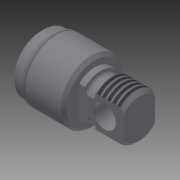
# Autodesk Inventor part: D-15705rear_head
Saved by Autodesk Inventor 2014 (Build 180170000, 170)
## iProperties
Created: 2014-01-19
Part Number: D-15705rear_head
Material: Steel
Catalog Web Link: www.cadenas.de
Description: Rear Head Cyl-Original Line Cyl
Vendor: BIMBA
Document SubType Name: Standard Catalog Part
Designer: Michael
Manufacturer: BIMBA
Density: 7.85 g/cm^3
Appearance: Steel
Mass: 19.7637 g
Surface Area: 18.1502 cm^2
Volume: 2.51767 cm^3
Category: PARTsolutions
Company: BIMBA
PSOL_IDENT_0: {$CADENAS_DATA\23d-libs\bimba\bimba\bimba_imperial\bimba_full_line\original_line_cylinders\three_pos
PSOL_IDENT_1: ition_cylinders\rear_head_cyl.prj},185 {VTYP=3D},{NB=D-15705rear_head},{LINA=D-15705rear_head},{NN=R
PSOL_IDENT_2: ear Head Cyl},{DATE=20.08.2011 07:16:50},{GEOMDATE=02.08.2011 10:58:00},{VERSION=},{LINEID=120},{LIN
PSOL_IDENT_3: ESUBID=-1},{WBVAR=Q,K}  {NB=D-15705rear_head},{LINA=D-15705rear_head},{KT=DUMMY},{PN=D-15705},{Q=},{
PSOL_IDENT_4: QALG= '' , 'Without Side Ported Rear Head' , 'Q' , 'With Side Ported Rear Head' },{K=},{KALG= '', 'S
PSOL_IDENT_5: tandard' , 'K' , 'Ports Rotated 90deg' },{TYPE=3},{ADDER=0.00000000},{A=0.53100000},{AA=0.12500000},
PSOL_IDENT_6: {A1=0.18800000},{A11=0.43800000},{A2=0.29700000},{A3=0.04000000},{A4=0.18500000},{A5=0.02500000},{A6=
PSOL_IDENT_7: 0.13200000},{A7=0.18500000},{A8=0.11200000},{B=0.61000000},{BB=0.49500000},{B1=0.52300000},{B2=0.573
PSOL_IDENT_8: 00000},{B3=0.37500000},{B4=0.31200000},{D=0.19000000},{DD=0.15900000},{CH=0.03000000},{CH1=0.0250000
PSOL_IDENT_9: 0},{CH2=0.03000000},{A111=1.15600000},{A55=0.02500000},{C=0.43700000},{C1=0.43200000},{C11=0.3070000
PSOL_IDENT_10: 0},{C2=0.78100000},{C21=0.78100000},{C22=0.78100000},{C3=0.15700000},{CCH=0.02000000},{CD=0.00000000
PSOL_IDENT_11: },{CDD=0.00000000},{RP=0.02185660},{NDM=0.43750},{CD1=0.43550},{CDD1=0.06000},{G=0.10000},{G1=0.0390
PSOL_IDENT_12: 0},{G2=0.03150},{BD=0.21850000}
CNS_NN: Rear Head Cyl
CNS_NT: Original Line Cyl
CNS_NB: D-15705rear_head
CNS_NBSYN: $PN.$Q.$K.rear_head
CNS_LINA: D-15705rear_head
CNS_PN: D-15705
CNS_Q: Without Side Ported Rear Head
CNS_QALG: '' , 'Without Side Ported Rear Head' , 'Q' , 'With Side Ported Rear Head'
CNS_K: Standard
CNS_KALG: '', 'Standard' , 'K' , 'Ports Rotated 90deg'
CNS_TYPE: 3
CNS_ADDER: 0.00000000
CNS_A: 0.53100000
CNS_AA: 0.12500000
CNS_A1: 0.18800000
CNS_A11: 0.43800000
CNS_A2: 0.29700000
CNS_A3: 0.04000000
CNS_A4: 0.18500000
CNS_A5: 0.02500000
CNS_A6: 0.13200000
CNS_A7: 0.18500000
CNS_A8: 0.11200000
CNS_B: 0.61000000
CNS_BB: 0.49500000
CNS_B1: 0.52300000
CNS_B2: 0.57300000
CNS_B3: 0.37500000
CNS_B4: 0.31200000
CNS_D: 0.19000000
CNS_DD: 0.15900000
CNS_CH: 0.03000000
CNS_CH1: 0.02500000
CNS_CH2: 0.03000000
CNS_A111: 1.15600000
CNS_A55: 0.02500000
CNS_C: 0.43700000
CNS_C1: 0.43200000
CNS_C11: 0.30700000
CNS_C2: 0.78100000
CNS_C21: 0.78100000
CNS_C22: 0.78100000
CNS_C3: 0.15700000
CNS_CCH: 0.02000000
CNS_CD: 0.00000000
CNS_CDD: 0.00000000
CNS_RP: 0.02185660
CNS_NDM: 0.43750
CNS_CD1: 0.43550
CNS_CDD1: 0.06000
CNS_G: 0.10000
CNS_G1: 0.03900
CNS_G2: 0.03150
CNS_BD: 0.21850000
SUPPLIER: BIMBA
ARTICLENO: D-15705rear_head
BOMINFO: D-15705rear_head
CREATOR: CADENAS GmbH
Title: D-15705rear_head
Author: Cadenas PARTsolutions
Comments: Original Line Cyl
Autodesk Inventor part; units mm, degrees
sketch "Sketch_1" plane through (0, 0, 0) normal (0, 0, 1) x (1, 0, 0)
  line L0 (13.4874, 0) -> (0, 0)
  line L1 (0, 0) -> (0, 6.5151)
  line L2 (0, 6.5151) -> (0.762, 7.2771)
  line L3 (0.762, 7.2771) -> (2.7178, 7.2771)
  line L4 (2.7178, 7.2771) -> (3.3528, 6.6421)
  line L5 (3.3528, 6.6421) -> (3.9878, 6.6421)
  line L6 (3.9878, 6.6421) -> (3.9878, 7.747)
  line L7 (3.9878, 7.747) -> (12.7254, 7.747)
  line L8 (12.7254, 7.747) -> (13.4874, 6.985)
  line L9 (13.4874, 6.985) -> (13.4874, 0)
  line L10 (13.4874, 0) -> (0, 0)
  constraints: 22 end point
revolve "Revolution1" add sketch "Sketch_1" angle 360 about axis through (13.4874, 0, 0) along (1, 0, 0)
sketch "Sketch2" plane through (0, 0, 0) normal (-1, 0, 0) x (0, 0, 1)
  point P0 (0, 0)
hole "Hole1" at (0, 0, 0) direction (1, 0, 0) diameter 9.525 depth 4.7752 countersink diameter 11.049 countersink angle 90
sketch "Sketch_6" plane through (0, 0, 0) normal (0, 0, 1) x (1, 0, 0)
  line L0 (11.9616, 0) -> (0, 0)
  line L1 (0, 0) -> (0, 2.0193)
  line L2 (0, 2.0193) -> (11.1252, 2.0193)
  line L3 (11.1252, 2.0193) -> (11.9616, 0)
  line L4 (11.9616, 0) -> (0, 0)
  constraints: 10 end point
revolve "Revolution2" cut sketch "Sketch_6" angle 360 about axis through (11.9616, 0, 0) along (1, 0, 0)
sketch "Sketch_9" plane through (0, 0, 0) normal (0, 0, 1) x (1, 0, 0)
  line L0 (13.4874, 0) -> (-13.4874, 0)
  line L1 (3.2301, 7.747) -> (3.2301, 7.6628)
  line L2 (3.2301, 7.6628) -> (4.2508, 6.6421)
  line L3 (4.2508, 6.6421) -> (4.5382, 6.6421)
  line L4 (4.5382, 6.6421) -> (3.4333, 7.747)
  line L5 (3.4333, 7.747) -> (3.2301, 7.747)
  constraints: 12 end point
revolve "Revolution3" add sketch "Sketch_9" angle 360 about axis through (13.4874, 0, 0) along (1, 0, 0)
sketch "Sketch_23" plane through (0, 0, 0) normal (0, 0, 1) x (1, 0, 0)
  line L0 (15.0114, 0) -> (13.4874, 0)
  line L1 (13.4874, 0) -> (13.4874, 5.5309)
  line L2 (13.4874, 5.5309) -> (15.0114, 5.5309)
  line L3 (15.0114, 5.5309) -> (15.0114, 0)
  line L4 (15.0114, 0) -> (13.4874, 0)
  constraints: 10 end point
revolve "Revolution4" add sketch "Sketch_23" angle 360 about axis through (15.0114, 0, 0) along (1, 0, 0)
sketch "Sketch_12" plane through (0, 0, 0) normal (0, 0, 1) x (1, 0, 0)
  line L0 (24.5872, 0) -> (13.4874, 0)
  line L1 (15.0114, 0) -> (15.0114, 5.3658)
  arc A0 (15.0114, 5.3658) -> (15.8115, 4.5656) centre (15.8115, 5.3657) ccw
  line L2 (15.8115, 4.5656) -> (16.7513, 4.5656)
  arc A1 (16.7513, 4.5656) -> (17.5514, 5.3658) centre (16.7513, 5.3657) ccw
  line L3 (17.5514, 5.3658) -> (17.5514, 5.5563)
  line L4 (17.5514, 5.5563) -> (23.8316, 5.5563)
  line L5 (23.8316, 5.5563) -> (24.5872, 4.8006)
  line L6 (24.5872, 4.8006) -> (24.5872, 0)
  line L7 (24.5872, 0) -> (15.0114, 0)
  constraints: 16 end point, 4 point on circle, 2 centre point
revolve "Revolution5" add sketch "Sketch_12" angle 360 about axis through (24.5872, 0, 0) along (1, 0, 0)
thread "Thread1" size "7/16-20 UNF" class "2A" standard "ANSI Unified Screw Threads" full length
sketch "Sketch_13" plane through (24.5872, 0, 0) normal (1, 0, 0) x (0, 0, -1)
  line L0 (-7.7978, -21.9456) -> (7.7978, -21.9456)
  line L1 (7.7978, -21.9456) -> (7.7978, 21.9456)
  line L2 (7.7978, 21.9456) -> (-7.7978, 21.9456)
  line L3 (-7.7978, 21.9456) -> (-7.7978, -21.9456)
  line L4 (-3.8989, -10.9728) -> (3.8989, -10.9728)
  line L5 (3.8989, -10.9728) -> (3.8989, 10.9728)
  line L6 (3.8989, 10.9728) -> (-3.8989, 10.9728)
  line L7 (-3.8989, 10.9728) -> (-3.8989, -10.9728)
  constraints: 16 end point
extrude "Extrusion1" cut sketch "Sketch_13" against normal blind 11.0998
sketch "Sketch_21" plane through (0, 0, 0) normal (0, 1, 0) x (-1, 0, 0)
  line L0 (-19.8374, 5.4864) -> (-19.8374, -5.4864)
  line L1 (-19.8374, -5.4864) -> (-22.6123, -5.4864)
  line L2 (-22.6123, -5.4864) -> (-22.6123, 5.4864)
  line L3 (-22.6123, 5.4864) -> (-19.8374, 5.4864)
  line L4 (-19.8374, 5.4864) -> (-19.8374, -5.4864)
  constraints: 10 end point
revolve "Revolution6" cut sketch "Sketch_21" angle 360 about axis through (19.8374, 0, 5.4864) along (0, 0, 1)
sketch "Sketch_17" plane through (0, 0, 0) normal (0, 1, 0) x (-1, 0, 0)
  line L0 (-10.3124, 0) -> (-10.3124, -7.747)
  line L1 (-10.3124, -7.747) -> (-14.2748, -7.747)
  line L2 (-14.2748, -7.747) -> (-14.2748, -6.731)
  line L3 (-14.2748, -6.731) -> (-12.7254, -6.731)
  line L4 (-12.7254, -6.731) -> (-12.2961, -6.3017)
  line L5 (-12.2961, -6.3017) -> (-12.2961, 0)
  line L6 (-12.2961, 0) -> (-10.3124, 0)
  line L7 (-10.3124, 0) -> (-10.3124, -7.747)
  constraints: 16 end point
revolve "Revolution7" cut sketch "Sketch_17" angle 360 about axis through (10.3124, 0, 0) along (0, 0, 1)
thread "Thread2" size "10-32 UNF" class "2B" standard "ANSI Unified Screw Threads" length 4.2824
ref_plane "aa2_XY" through (19.8374, 0, 0) normal (0, 1, 0) x (1, 0, 0)
ref_plane "aa2_YZ" through (19.8374, 0, 0) normal (1, 0, 0) x (0, 0, -1)
ref_plane "aa2_ZX" through (19.8374, 0, 0) normal (0, 0, -1) x (0, 1, 0)
ref_plane "mm1_XY" through (10.3124, 0, 0) normal (0, 1, 0) x (1, 0, 0)
ref_plane "mm1_YZ" through (10.3124, 0, 0) normal (1, 0, 0) x (0, 0, -1)
ref_plane "mm1_ZX" through (10.3124, 0, 0) normal (0, 0, -1) x (0, 1, 0)
ref_plane "mm2_XY" through (19.8374, 0, 0) normal (0, 1, 0) x (1, 0, 0)
ref_plane "mm2_YZ" through (19.8374, 0, 0) normal (1, 0, 0) x (0, 0, -1)
ref_plane "mm2_ZX" through (19.8374, 0, 0) normal (0, 0, -1) x (0, 1, 0)
ref_plane "nn1_XY" through (24.5872, 0, 3.8989) normal (1, 0, 0) x (0, 0, -1)
ref_plane "nn1_YZ" through (24.5872, 0, 3.8989) normal (0, 0, -1) x (0, 1, 0)
ref_plane "nn1_ZX" through (24.5872, 0, 3.8989) normal (0, 1, 0) x (1, 0, 0)
ref_plane "nn2_XY" through (24.5872, 0, -3.8989) normal (1, 0, 0) x (0, 0, -1)
ref_plane "nn2_YZ" through (24.5872, 0, -3.8989) normal (0, 0, -1) x (0, 1, 0)
ref_plane "nn2_ZX" through (24.5872, 0, -3.8989) normal (0, 1, 0) x (1, 0, 0)
ref_plane "p1_XY" through (13.4874, 0, 0) normal (0, 1, 0) x (1, 0, 0)
ref_plane "p1_YZ" through (13.4874, 0, 0) normal (1, 0, 0) x (0, 0, -1)
ref_plane "p1_ZX" through (13.4874, 0, 0) normal (0, 0, -1) x (0, 1, 0)
ref_plane "q2_XY" through (24.5872, 0, 0) normal (0, 1, 0) x (1, 0, 0)
ref_plane "q2_YZ" through (24.5872, 0, 0) normal (1, 0, 0) x (0, 0, -1)
ref_plane "q2_ZX" through (24.5872, 0, 0) normal (0, 0, -1) x (0, 1, 0)
ref_plane "r1_XY" through (17.8435, 0, 0) normal (0, 1, 0) x (1, 0, 0)
ref_plane "r1_YZ" through (17.8435, 0, 0) normal (1, 0, 0) x (0, 0, -1)
ref_plane "r1_ZX" through (17.8435, 0, 0) normal (0, 0, -1) x (0, 1, 0)
ref_plane "r2_XY" through (21.8313, 0, 0) normal (0, 1, 0) x (1, 0, 0)
ref_plane "r2_YZ" through (21.8313, 0, 0) normal (1, 0, 0) x (0, 0, -1)
ref_plane "r2_ZX" through (21.8313, 0, 0) normal (0, 0, -1) x (0, 1, 0)
ref_plane "rear_head_XY" through (2.7178, 0, 0) normal (1, 0, 0) x (0, 0, -1)
ref_plane "rear_head_YZ" through (2.7178, 0, 0) normal (0, 0, -1) x (0, 1, 0)
ref_plane "rear_head_ZX" through (2.7178, 0, 0) normal (0, 1, 0) x (1, 0, 0)
ref_plane "to_bushing_XY" through (19.8374, 0, 0) normal (0, 0, 1) x (1, 0, 0)
ref_plane "to_bushing_YZ" through (19.8374, 0, 0) normal (1, 0, 0) x (0, 1, 0)
ref_plane "to_bushing_ZX" through (19.8374, 0, 0) normal (0, 1, 0) x (0, 0, 1)
ref_plane "to_mounting_bracket_xp_XY" through (13.4874, 0, 0) normal (1, 0, 0) x (0, 0, -1)
ref_plane "to_mounting_bracket_xp_YZ" through (13.4874, 0, 0) normal (0, 0, -1) x (0, 1, 0)
ref_plane "to_mounting_bracket_xp_ZX" through (13.4874, 0, 0) normal (0, 1, 0) x (1, 0, 0)
ref_plane "to_pivot_bracket_XY" through (19.8374, 0, 0) normal (0, 0, 1) x (1, 0, 0)
ref_plane "to_pivot_bracket_YZ" through (19.8374, 0, 0) normal (1, 0, 0) x (0, 1, 0)
ref_plane "to_pivot_bracket_ZX" through (19.8374, 0, 0) normal (0, 1, 0) x (0, 0, 1)
body "Solid1"
